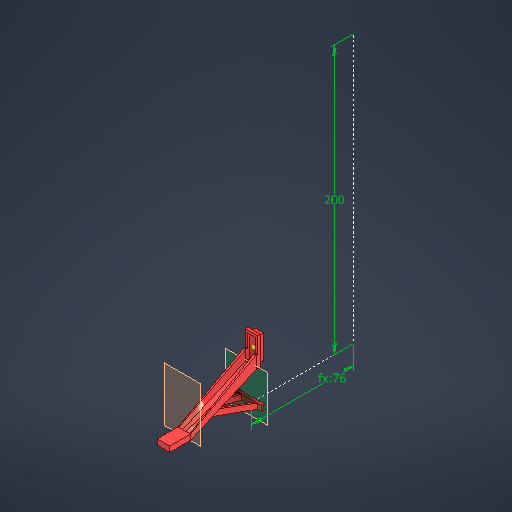
# Autodesk Inventor part: load_cell_holder_1
Saved by Autodesk Inventor 2026 (Build 300175000, 175)
## iProperties
Created: 2025-05-06
Part Number: load_cell_holder_1
Material: Generic
Document SubType Name: Modeling
Designer: Paul Juschitz
Density: 1 g/cm^3
Appearance: Light Red
Author: Paul Juschitz
Autodesk Inventor part; units mm, degrees
ref_plane "YZ Plane" through (0, 0, 0) normal (1, 0, 0) x (0, 1, 0)
ref_plane "XZ Plane" through (0, 0, 0) normal (0, 1, 0) x (-1, 0, 0)
ref_plane "XY Plane" through (0, 0, 0) normal (0, 0, 1) x (1, 0, 0)
sketch "Sketch1" plane through (0, 0, 0) normal (0, 0, 1) x (1, 0, 0)
  line L0 (-3.05, 8.75) -> (3.05, 8.75)
  line L1 (3.05, 8.75) -> (3.05, -8.75)
  line L2 (3.05, -8.75) -> (-3.05, -8.75)
  line L3 (-3.05, -8.75) -> (-3.05, 8.75)
  line L4 (-3.05, 8.75) -> (3.05, -8.75) construction
  line L5 (3.05, 8.75) -> (-3.05, -8.75) construction
  point P0 (0, 0)
  dimension "d0" = 6.1
  dimension "d1" = 17.5
  constraints: 12 end point, 2 midpoint, 2 parallel, 1 horizontal, 1 perpendicular
  measures "d0" distance of L1.end L2.end
  measures "d1" distance of L0.end L1.end
extrude "Extrusion1" add sketch "Sketch1" against normal blind 4
sketch "Sketch2" plane through (0, 0, 0) normal (0, 0, 1) x (1, 0, 0)
  line L0 (-3.05, 8.75) -> (3.05, 8.75) projected
  line L1 (0, 8.75) -> (0, -8.75) construction
  line L2 (3.05, -8.75) -> (-3.05, -8.75) projected
  line L3 (3.05, 8.75) -> (3.05, -8.75) projected
  line L4 (3.05, 0) -> (-3.05, 0) construction
  line L5 (-3.05, -8.75) -> (-3.05, 8.75) projected
  line L6 (-4.55, 10.75) -> (4.55, 10.75)
  line L7 (4.55, 10.75) -> (4.55, -10.75)
  line L8 (4.55, -10.75) -> (-4.55, -10.75)
  line L9 (-4.55, -10.75) -> (-4.55, 10.75)
  line L10 (-4.55, 10.75) -> (4.55, -10.75) construction
  line L11 (4.55, 10.75) -> (-4.55, -10.75) construction
  point P0 (0, 0)
  dimension "d4" = 2
  dimension "d5" = 1.5
  constraints: 16 end point, 6 midpoint, 2 parallel, 1 horizontal, 1 perpendicular
  measures "d4" distance between parallel lines of L8 L2
  measures "d5" distance between parallel lines of L3 L7
extrude "Extrusion2" add sketch "Sketch2" along normal blind 2
ref_plane "Work Plane1" through (0, 0, 52) normal (0, 0, 1) x (1, 0, 0)
sketch "Sketch3" plane through (0, 0, 52) normal (0, 0, 1) x (1, 0, 0)
  line L0 (-4.55, -10.75) -> (4.55, -10.75)
  line L1 (0, -10.75) -> (0, -59.663767)
  line L2 (-4.66, -27.75) -> (4.66, -27.75)
  line L3 (4.66, -27.75) -> (4.66, -31.75)
  line L4 (4.66, -31.75) -> (-4.66, -31.75)
  line L5 (-4.66, -31.75) -> (-4.66, -27.75)
  line L6 (-4.66, -27.75) -> (4.66, -31.75) construction
  line L7 (4.66, -27.75) -> (-4.66, -31.75) construction
  point P0 (0, 0)
  point P1 (0, -29.75)
  dimension "d9" = 9.32
  dimension "d10" = 4
  dimension "load_cell_holder_setdown" = 17
  constraints: 14 end point, 3 midpoint, 2 parallel, 1 horizontal, 1 perpendicular, 1 point on line, 1 vertical
  measures "d9" distance of L3.end L4.end
  measures "d10" distance between parallel lines of L2 L4
  measures "load_cell_holder_setdown" distance between parallel lines of L0 L2
extrude "Extrusion3" add sketch "Sketch3" along normal blind 15.48
sketch "Sketch4" plane through (0, 0, 2) normal (0, 0, 1) x (1, 0, 0)
  line L0 (-4.55, -10.75) -> (4.55, -10.75) projected
  line L1 (-4.55, -10.75) -> (4.55, -10.75)
  line L2 (4.55, -10.75) -> (4.55, -1.25)
  line L3 (4.55, -1.25) -> (3.05, -1.25)
  line L4 (3.05, -8.75) -> (-3.05, -8.75) projected
  line L5 (3.05, -8.75) -> (-3.05, -8.75)
  line L6 (-3.05, -8.75) -> (-3.05, -1.25)
  line L7 (-3.05, -1.25) -> (-4.55, -1.25)
  line L8 (-4.55, -1.25) -> (-4.55, -10.75)
  line L9 (3.05, -1.25) -> (3.05, -8.75)
  line L10 (4.55, -10.75) -> (4.55, 10.75) projected
  line L11 (3.05, 8.75) -> (3.05, -8.75) projected
  line L12 (3.05, -8.75) -> (-3.05, -8.75) projected
  dimension "d15" = 9.5
  constraints: 16 end point, 6 perpendicular, 2 collinear, 2 point on line
  measures "d15" distance of L0.end L2.end
extrude "Extrusion4" add sketch "Sketch4" along normal blind 1
loft "Loft1" add section 1 edges at (0, -10.75, 3) (4.55, -6, 3) (3.8, -1.25, 3) (3.05, -5, 3) (0, -8.75, 3) (-3.05, -5, 3) (-3.8, -1.25, 3) (-4.55, -6, 3) section 2 edges at (0, -31.75, 52) (-4.66, -29.75, 52) (0, -27.75, 52) (4.66, -29.75, 52)
sketch "Sketch5" plane through (-4.66, -31.75, 52) normal (0, -0.919145, -0.3939193) x (1, 0, 0)
  line L0 (0.11, -53.310412) -> (0, 0) construction
  line L1 (0.037141, -18) -> (1.537141, -18)
  line L2 (1.537141, -18) -> (1.537141, -24)
  line L3 (1.537141, -24) -> (0.037141, -24)
  line L4 (0.037141, -24) -> (0.037141, -18)
  line L5 (0, 0) -> (9.32, 0) construction
  point P0 (4.66, -60.302479)
  point P1 (0.787141, -18)
  dimension "d22" = 1.5
  dimension "d23" = 6
  dimension "d24" = 18
  constraints: 8 end point, 2 parallel, 1 horizontal, 1 midpoint, 1 perpendicular, 1 point on line
  measures "d22" distance of L2.end L3.end
  measures "d23" distance between parallel lines of L1 L3
  measures "d24" distance from line of point (0.787, -18) L5
ref_plane "Work Plane2" through (0, 0, 4) normal (0, 0, -1) x (-1, 0, 0)
sketch "Sketch6" plane through (0, 0, 4) normal (0, 0, -1) x (-1, 0, 0)
  line L0 (3.05, -8.75) -> (-3.05, -8.75) construction
  line L1 (6.5, -30.75) -> (5, -30.75)
  line L2 (5, -30.75) -> (5, -34.75)
  line L3 (5, -34.75) -> (6.5, -34.75)
  line L4 (6.5, -34.75) -> (6.5, -30.75)
  line L5 (0, -8.75) -> (0, -58.75)
  point P0 (0, 0)
  point P1 (5.75, -30.75)
  dimension "d26" = 1.5
  dimension "d27" = 4
  dimension "cell_holder_foot_setdown" = 22
  dimension "d29" = 50
  dimension "cell_holder_foot_setout" = 10
  constraints: 10 end point, 2 midpoint, 2 parallel, 1 horizontal, 1 perpendicular, 1 vertical
  measures "d26" distance of L3.end L2.end
  measures "d27" distance of L2.end L1.end
  measures "cell_holder_foot_setdown" distance from line of point (5.75, -30.75) L0
  measures "d29" distance of L5.start L5.end
  measures "cell_holder_foot_setout" diameter of L2 L5
loft "Loft2" add profiles "Sketch5", "Sketch6"
mirror "Mirror1" about plane through (0, 0, 0) normal (1, 0, 0) of "Loft2"
sketch "Sketch7" plane through (0, 0, 4) normal (0, 0, -1) x (-1, 0, 0)
  line L0 (-9.5, -30.75) -> (9.5, -30.75)
  line L1 (9.5, -30.75) -> (9.5, -34.75)
  line L2 (9.5, -34.75) -> (-9.5, -34.75)
  line L3 (-9.5, -34.75) -> (-9.5, -30.75)
  line L4 (4.55, -10.75) -> (-4.55, -10.75)
  line L5 (0, -10.75) -> (0, -43.204037)
  point P0 (0, 0)
  point P1 (-6.5, -30.75)
  point P2 (6.5, -30.75)
  point P3 (6.5, -34.75)
  point P4 (-6.5, -34.75)
  dimension "d36" = 3
  constraints: 10 end point, 2 parallel, 2 point on line, 1 horizontal, 1 midpoint, 1 perpendicular, 1 vertical, 1 other
  measures "d36" distance from line of point (-6.5, -30.75) L3
extrude "Extrusion6" add sketch "Sketch7" along normal blind 1
sketch "Sketch10" plane through (0, 0, 0) normal (1, 0, 0) x (0, 1, 0)
  line L0 (-34.75, 2) -> (-34.75, -74) construction
  line L1 (-34.75, -74) -> (165.25, -74) construction
  point P0 (0, 0)
  dimension "d45" = 76
  dimension "d46" = 200
  constraints: 4 end point, 1 horizontal, 1 vertical
  measures "d45" distance of L0.start L0.end
  measures "d46" distance of L0.end L1.end
sketch "Sketch11" plane through (0, 0, 3) normal (0, 0, -1) x (-1, 0, 0)
  line L0 (-9.5, -34.75) -> (9.5, -34.75) projected
  line L1 (9.5, -34.75) -> (9.5, -30.75) projected
  line L2 (9.5, -30.75) -> (-9.5, -30.75) projected
  line L3 (-9.5, -30.75) -> (-9.5, -34.75) projected
  point P0 (0, 0)
extrude "Extrusion7" add sketch "Sketch11" along normal blind 2
sketch "Sketch12" plane through (0, 0, 0) normal (1, 0, 0) x (0, 1, 0)
  line L0 (-30.75, 1) -> (-34.75, 1)
  line L1 (-30.75, 1) -> (-30.75, 2.2)
  line L2 (-30.75, 1) -> (-34.75, 1)
  line L3 (-34.75, 1) -> (-34.75, 3.3)
  arc A0 (-30.75, 2.2) -> (-34.75, 3.3) centre (-34.280362, -2.814952) ccw
  point P0 (0, 0)
  dimension "d49" = 1.2
  dimension "d50" = 2.3
  dimension "d51" = 6.13296
  constraints: 6 end point, 2 point on circle, 1 centre point, 1 perpendicular, 1 vertical
  measures "d49" distance of L0.start L1.end
  measures "d50" distance of L0.end L3.end
  measures "d51" radius of A0
revolve "Revolution2" cut sketch "Sketch12" angle 180 mid plane about axis through (0, -34.75, -74) along (0, 1, 0)
equation "\"d1\" = 0.5 * m2m_fork_opening_height"
equation "\"d9\" = load_cell_width"
equation "\"d45\" = m2m_bottom_radius_lower"
equation "\"m2m_fork_opening_height\" = 35"
equation "\"load_cell_width\" = 9.32"
equation "\"m2m_bottom_radius_lower\" = 76"
body "Solid1"
